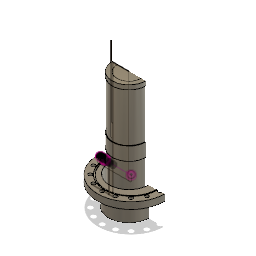
low vibration interface cryo v11 (Autodesk Fusion 360 archive; units mm, degrees)
design "low vibration interface cryo" references "CF100 profile"
Autodesk Fusion 360 part; units mm, degrees
derive "ExternalDerived1" from "CF100 profile v1"
sketch "Sketch1" plane through (0, 0, 0) normal (0, 0, 1) x (1, 0, 0)
  line L0 (-57.4316, -1.2) -> (0, -1.2)
  line L1 (-57.65, -0.6) -> (-57.4316, -1.2)
  line L2 (-60.35, -1.5827) -> (-57.65, -0.6)
  line L3 (-60.35, 0) -> (-60.35, -1.5827)
  line L4 (-60.35, 0) -> (-69.35, 0)
  line L5 (-69.35, 0) -> (-75.8, 0)
  line L6 (-75.8, 0) -> (-75.8, -15)
  line L7 (-75.8, -15) -> (0, -15)
  line L8 (0, -15) -> (0, 0)
  line L9 (-65.15, 0) -> (-65.15, -15)
  line L10 (-60.95, 0) -> (-60.95, -15)
  line L11 (-69.35, 0) -> (-69.35, -15)
  line L12 (-43, 200) -> (-5, 200)
  line L13 (-5, 200) -> (-5, -15)
  line L14 (-5, 199) -> (-32, 199)
  line L15 (-32, 199) -> (-32, 198)
  line L16 (-32, 198) -> (-41, 198)
  line L17 (-41.5, 190) -> (-41.5, 80)
  line L18 (-41.5, 80) -> (-43, 80)
  line L19 (-43, 80) -> (-43, 50)
  line L20 (-43, 50) -> (-41.5, 50)
  line L21 (-41.5, 50) -> (-41.5, -55)
  line L22 (-43, 200) -> (-43, 190)
  line L23 (-43, 190) -> (-41.5, 190)
  line L24 (-41, 198) -> (-41, -1.2)
  line L25 (-41.5, -55) -> (-43, -55)
  line L26 (-43, -55) -> (-43, -63)
  line L27 (-41, -1.2) -> (-41, -15)
  line L28 (-41, -15) -> (-41, -65)
  line L29 (-51, -65) -> (-41, -65)
  line L30 (-51, -65) -> (-51, -1.2)
  line L31 (-49, -1.2) -> (-49, -63)
  line L32 (-49, -63) -> (-43, -63)
  line L33 (-49, -63) -> (-90, -63)
  line L34 (-90, -63) -> (-90, -65)
  line L35 (-90, -65) -> (-51, -65)
  line L36 (-43, 50) -> (-46, 50)
  line L37 (-46, 50) -> (-46, 240)
  line L38 (-46, 240) -> (-44.5, 240)
  line L39 (-44.5, 240) -> (-44.5, 80)
  line L40 (-44.5, 80) -> (-43, 80)
  dimension "d1" = 75.8
  dimension "d2" = 15
  dimension "d4" = 200
  dimension "d8" = 2
  dimension "d9" = 1
  dimension "d11" = 2
  dimension "d12" = 0.5
  dimension "d13" = 10
  dimension "d14" = 38
  dimension "d17" = 30
  dimension "d18" = 9
  dimension "d23" = 10
  dimension "d24" = 2
  dimension "d25" = 50
  dimension "d26" = 2
  dimension "d27" = 10
  dimension "d28" = 50
  dimension "d29" = 90
  dimension "d30" = 5
  dimension "d33" = 3
  dimension "d34" = 1.5
  dimension "d35" = 40
  measures "d2" distance of L5 L7
  measures "d4" distance of L5 L12
  measures "d8" distance of L12 L16
  measures "d9" distance of L12 L14
  measures "d11" distance of L22 L24
  measures "d12" distance of L17 L24
  measures "d13" distance of L12 L23
  measures "d14" distance of L13 L22
  measures "d17" distance of L18 L20
  measures "d18" distance of L15 L24
  measures "d23" distance of L25 L29
  measures "d24" distance of L29 L32
  measures "d25" distance of L7 L29
  measures "d27" distance of L28 L30
  measures "d28" distance of L5 L20
  measures "d29" distance of L8 L34
  measures "d30" distance of L8 L13
  measures "d33" distance of L19 L37
  measures "d34" distance of L19 L39
  measures "d35" distance of L12 L38
revolve "Revolve1" add sketch "Sketch1" angle 360 about axis through (0, -15, 0) along (0, 1, 0) contours L0 L1 L2 L3 L4 L7 L10 L30 | L0 L7 L30 L31 | L0 L7 L21 L31 | L0 L7 L21 L27 | L4 L7 L9 L10 | L0 L7 L13 L27 | L4 L7 L9 L11 | L0 L7 L8 L13 | L5 L6 L7 L11 makes body 1
revolve "Revolve2" cut sketch "Sketch1" angle 360 about axis through (-65.15, 0, 0) along (0, -1, 0) contours L4 L7 L9 L10 bodies 1
pattern_circular "C-Pattern1" count 16 over 360 about axis through (0, 1.75, 0) along (0, 1, 0) of "Revolve2"
revolve "Revolve3" cut sketch "Sketch1" angle 360 about axis through (-5, 200, 0) along (0, -1, 0) contours L0 L7 L21 L31 | L0 L7 L21 L27 | L0 L7 L13 L27 bodies 1
revolve "Revolve4" add sketch "Sketch1" angle 360 about axis through (-5, 200, 0) along (0, -1, 0) contours L7 L30 L31 L33 | L0 L12 L13 L14 L15 L16 L17 L18 L19 L20 L21 L22 L23 L24 | L0 L7 L21 L27 | L7 L21 L25 L26 L28 L29 L30 L32 L33 bodies 1
revolve "Revolve5" add sketch "Sketch1" angle 360 about axis through (-5, 200, 0) along (0, -1, 0) separate body contours L19 L36 L37 L38 L39 L40 makes body 2
hidden bodies 2
equation "d1 = ( 151.6 / 2 ) * 1 mm"
equation "d29 = ( 180 / 2 ) * 1 mm"
named bodies: "lov vibration interface", "thermal shield"
